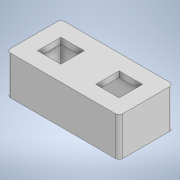
# Autodesk Inventor part: Keyboard_Base
Saved by Autodesk Inventor 2021 (Build 250183000, 183)
## iProperties
Created: 2020-07-07
Part Number: Keyboard_Base
Material: Generic
Document SubType Name: Modeling
Designer: ameli
Density: 1 g/cm^3
Appearance: Default
Author: ameli
Autodesk Inventor part; units mm, degrees
ref_plane "YZ Plane" through (0, 0, 0) normal (1, 0, 0) x (0, 1, 0)
ref_plane "XZ Plane" through (0, 0, 0) normal (0, 1, 0) x (-1, 0, 0)
ref_plane "XY Plane" through (0, 0, 0) normal (0, 0, 1) x (1, 0, 0)
sketch "Sketch1" plane through (0, 0, 0) normal (0, 1, 0) x (-1, 0, 0)
  line L0 (14.5, 7) -> (-14.5, 7)
  line L1 (-14.5, 7) -> (-14.5, -7)
  line L2 (-14.5, -7) -> (14.5, -7)
  line L3 (14.5, -7) -> (14.5, 7)
  point P0 (0, 0)
  dimension "d0" = 14
  dimension "d1" = 29
  dimension "d2" = 14.5
  dimension "d3" = 7
  constraints: 8 end point, 2 parallel, 1 horizontal, 1 perpendicular
  measures "d0" distance of L2.end L0.start
  measures "d1" distance of L1.end L2.end
  measures "d2" distance from line of point (0, 0) L3
  measures "d3" distance from line of point (0, 0) L2
extrude "Extrusion1" add sketch "Sketch1" along normal blind 10
fillet "Fillet1" radius 1 4 edges at (14.5, 5, 7) (14.5, 5, -7) (-14.5, 5, -7) (-14.5, 5, 7)
shell "Shell1" thickness 1.5 removed faces 1 at (4.5, 0, 2.3333)
sketch "Sketch3" plane through (0, 10, 0) normal (0, 1, 0) x (1, 0, 0)
  line L0 (-10.5, -3) -> (-4.5, -3)
  line L1 (-4.5, -3) -> (-4.5, 3)
  line L2 (-4.5, 3) -> (-10.5, 3)
  line L3 (-10.5, 3) -> (-10.5, -3)
  line L4 (4.5, -3) -> (10.5, -3)
  line L5 (10.5, -3) -> (10.5, 3)
  line L6 (10.5, 3) -> (4.5, 3)
  line L7 (4.5, 3) -> (4.5, -3)
  line L8 (-13.5, -7) -> (13.5, -7) projected
  line L9 (-14.5, 6) -> (-14.5, -6) projected
  line L10 (14.5, -6) -> (14.5, 6) projected
  point P0 (0, 0)
  dimension "d14" = 6
  dimension "d15" = 6
  dimension "d16" = 4
  dimension "d17" = 4
  dimension "d18" = 4
  dimension "d19" = 6
  constraints: 16 end point, 4 parallel, 2 horizontal, 2 perpendicular, 2 point on line
  measures "d14" distance of L2.end L0.start
  measures "d15" distance of L1.end L2.end
  measures "d16" distance between parallel lines of L8 L0
  measures "d17" distance between parallel lines of L9 L3
  measures "d18" distance between parallel lines of L10 L5
  measures "d19" distance of L5.end L6.end
extrude "Extrusion3" cut sketch "Sketch3" against normal through all
body "Solid1"
